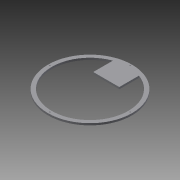
# Autodesk Inventor part: Base_Acryllic
Saved by Autodesk Inventor 2015 SP1 (Build 190203100, 203)
## iProperties
Created: 2016-03-29
Part Number: Base_Acryllic
Material: Generic
Document SubType Name: Modeling
Designer: Ethan
Density: 1 g/cm^3
Appearance: Default
Author: Ethan
Autodesk Inventor part; units mm, degrees
ref_plane "YZ Plane" through (0, 0, 0) normal (1, 0, 0) x (0, 1, 0)
ref_plane "XZ Plane" through (0, 0, 0) normal (0, 1, 0) x (-1, 0, 0)
ref_plane "XY Plane" through (0, 0, 0) normal (0, 0, 1) x (1, 0, 0)
sketch "Sketch1" plane through (0, 0, 0) normal (0, 1, 0) x (-1, 0, 0)
  circle A0 centre (0, 0) radius 139.7
  circle A1 centre (0, 133.35) radius 1.5875
  circle A2 centre (-133.35, 0) radius 1.5875
  circle A3 centre (0, -133.35) radius 1.5875
  circle A4 centre (133.35, 0) radius 1.5875
  arc A5 (43.2777, -119.3986) -> (-43.2777, -119.3986) centre (0, 0) ccw
  line L0 (43.2777, -54.0192) -> (-43.2777, -54.0192)
  line L1 (-43.2777, -54.0192) -> (-43.2777, -119.3986)
  line L2 (0, -97.1997) -> (0, -97.2112)
  line L3 (43.2777, -119.3986) -> (43.2777, -54.0192)
  dimension "d0" = 279.4
  dimension "d97" = 3.175
  dimension "d100" = 360
  dimension "d131" = 254
  constraints: 8 end point, 6 centre point, 2 coincident, 2 point on circle, 1 parallel, 1 perpendicular, 9 other
  measures "d0" diameter of A0
  measures "d97" diameter of A1
  measures "d131" diameter of A5
extrude "Extrusion10" add sketch "Sketch1" along normal blind 6.35
body "Solid8"
